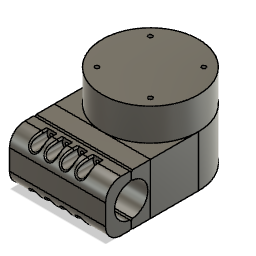
LIDAR Model Stand (Autodesk Fusion 360 design; units mm, degrees)
Autodesk Fusion 360 part; units mm, degrees
box "BoxPrimitive1" add length 75 width 75 height 55 placed x (0, 1, 0) y (-1, 0, 0) z (0, 0, 1) at (70, 0, 0) makes body 1
move_face "OffsetFaces3" offset -15 1 faces at (20, 25, 0) on bodies 1
sketch "Sketch4" plane through (0, 0, 0) normal (1, 0, 0) x (0, 0, -1)
  circle A0 centre (-35, -15) radius 13
  circle A1 centre (-35, -15) radius 20
  line L0 (-55, 0) -> (-55, -15)
  line L1 (-15.0241, -0.1224) -> (-15, -15)
  line L2 (-55, -15) -> (-15, -15)
  line L3 (-15.0241, -0.1224) -> (-55, 0)
  point P0 (-55, 0)
  dimension "d13" = 26
  dimension "d14" = 40
  constraint concentric A0 A1
  constraint vertical L0
  constraint coincident A1 L0.end
  constraint tangent A1 L0
  constraint coincident A1 L1.end
  constraint perpendicular L0 L2
  measures "d13" diameter of A0
  measures "d14" diameter of A1
extrude "Extrude3" add sketch "Sketch4" along normal blind 70 contours A1 L1 L3 | A0 A1 L2 L3 | A1 L0 L3 bodies 1
sketch "Sketch5" plane through (0, -15, 0) normal (0, -1, 0) x (1, 0, 0)
  line L0 (0, 55) -> (0, 48)
  line L1 (0, 48) -> (70, 48)
  line L2 (70, 48) -> (70, 55)
  line L3 (70, 55) -> (0, 55)
  line L4 (0, 51.5) -> (70, 51.5) construction
  circle A0 centre (12, 51.5) radius 1.1
  circle A1 centre (24, 51.5) radius 1.1
  circle A2 centre (36, 51.5) radius 1.1
  circle A3 centre (48, 51.5) radius 1.1
  line L5 (0, 48) -> (60, 48)
  line L6 (60, 48) -> (60, 35)
  line L7 (60, 35) -> (0, 35)
  line L8 (0, 35) -> (0, 48)
  circle A4 centre (12, 18.5) radius 1.1
  circle A5 centre (24, 18.5) radius 1.1
  circle A6 centre (36, 18.5) radius 1.1
  circle A7 centre (48, 18.5) radius 1.1
  dimension "d18" = 12
  dimension "d19" = 12
  dimension "d20" = 12
  dimension "d21" = 12
  dimension "d22" = 2.2
  dimension "d23" = 60
  dimension "d24" = 13
  constraint midpoint L0 L4.start
  constraint midpoint L2 L4.end
  constraint coincident L4 A0.centre
  constraint coincident L4 A1.centre
  constraint coincident L4 A2.centre
  constraint coincident L4 A3.centre
  constraint equal A1 A2
  constraint equal A2 A3
  constraint equal A0 A1
  constraint horizontal L5
  constraint vertical L6
  constraint horizontal L7
  constraint vertical L8
  constraint coincident L0.end L1.start
  constraint symmetric A0 L7 A4
  constraint symmetric A1 L7 A5
  constraint symmetric A2 L7 A6
  constraint symmetric A3 L7 A7
  measures "d18" distance of L4.start A0.centre
  measures "d19" distance of A0.centre A1.centre
  measures "d20" distance of A1.centre A2.centre
  measures "d21" distance of A2.centre A3.centre
  measures "d22" diameter of A0
  measures "d23" distance of L0.end L5.end
  measures "d24" distance of L0.end L7.end
extrude "Extrude4" cut sketch "Sketch5" against normal blind 15 contours A0 | A1 | A2 | A3 | A4 | A5 | A6 | A7 bodies 1
chamfer "Chamfer1" distance 1 angle 45 3 edges at (35, -15, 22) (35, -15, 48) (35, -15, 55) on bodies 1
sketch "Sketch6" plane through (0, 0, 0) normal (-1, 0, 0) x (0, 0, 1)
  line L0 (15.0241, -0.1224) -> (15, -15)
  line L1 (15, -15) -> (21, -15)
  line L2 (21, -15) -> (22.0385, -14.0007)
  arc A0 (47.9615, -14.0007) -> (22.0385, -14.0007) centre (35, -15) ccw
  line L3 (47.9615, -14.0007) -> (49, -15)
  line L4 (49, -15) -> (54, -15)
  circle A1 centre (35, -15) radius 13
  circle A2 centre (35, -15) radius 20
  line L5 (15, -15) -> (55, -15)
  line L6 (55, -15) -> (55, -23)
  line L7 (43, -35) -> (27, -35)
  line L8 (15, -23) -> (15, -15)
  arc A3 (15, -23) -> (27, -35) centre (27, -23) ccw
  arc A4 (43, -35) -> (55, -23) centre (43, -23) ccw
  line L9 (54, -15) -> (55, -14)
  line L10 (55, -14) -> (55, 0)
  line L11 (55, 0) -> (15.0241, -0.1224)
  dimension "d29" = 40
  dimension "d30" = 12
  constraint concentric A0 A1
  constraint coincident A0.start A1
  constraint concentric A1 A2
  constraint horizontal L5
  constraint vertical L6
  constraint horizontal L7
  constraint vertical L8
  constraint coincident L0.end L1.start
  constraint tangent A2 L6
  constraint tangent A2 L7
  constraint tangent L7 A3
  constraint tangent L8 A3
  constraint tangent L6 A4
  constraint tangent L7 A4
  constraint equal A3 A4
  measures "d29" diameter of A2
  measures "d30" radius of A3
extrude "Extrude5" add sketch "Sketch6" against normal blind 70 separate body contours L1 L4 A1 A2 L5 | A2 L7 L8 A3 | A2 L6 L7 A4 makes body 2
chamfer "Chamfer3" distance 1 angle 45 4 edges at (35, -15, 22) (35, -15, 55) (35, -15, 48) (35, -15, 15) on bodies 2
chamfer "Chamfer4" distance 1 angle 45 1 edges at (35, -15, 15) on bodies 1
sketch "Sketch7" plane through (0, -15, 0) normal (0, -1, 0) x (1, 0, 0)
  circle A0 centre (24, 51.5) radius 1.1
  circle A1 centre (36, 51.5) radius 1.1
  circle A2 centre (12, 51.5) radius 1.1
  circle A3 centre (48, 51.5) radius 1.1
  line L0 (70, 54) -> (0, 54)
  line L1 (0, 54) -> (0, 49)
  line L2 (0, 49) -> (70, 49)
  line L3 (70, 49) -> (70, 54)
sketch "Sketch8" plane through (0, -15, 0) normal (0, -1, 0) x (1, 0, 0)
  circle A0 centre (36, 18.5) radius 1.1
  circle A1 centre (24, 18.5) radius 1.1
  circle A2 centre (48, 18.5) radius 1.1
  circle A3 centre (12, 18.5) radius 1.1
  line L0 (0, 16) -> (70, 16)
  line L1 (70, 16) -> (70, 21)
  line L2 (70, 21) -> (0, 21)
  line L3 (0, 21) -> (0, 16)
extrude "Extrude6" cut sketch "Sketch8" sketch "Sketch7" along normal blind 23 contours A0 | A1 | A2 | A3 of sketch 2 contours A0 | A1 | A2 | A3 bodies 2
sketch "Sketch9" plane through (0, -15, 0) normal (0, 1, 0) x (-1, 0, 0)
  circle A0 centre (-24, 51.5) radius 1.1
  circle A1 centre (-36, 51.5) radius 1.1
  circle A2 centre (-12, 51.5) radius 1.1
  circle A3 centre (-48, 51.5) radius 1.1
  line L0 (-70, 49) -> (0, 49)
  line L1 (0, 49) -> (0, 54)
  line L2 (0, 54) -> (-70, 54)
  line L3 (-70, 54) -> (-70, 49)
  circle A4 centre (-12, 51.5) radius 3.75
  circle A5 centre (-24, 51.5) radius 3.75
  circle A6 centre (-36, 51.5) radius 3.75
  circle A7 centre (-48, 51.5) radius 3.75
  circle A8 centre (-12, 18.5) radius 3.75
  circle A9 centre (-24, 18.5) radius 3.75
  circle A10 centre (-36, 18.5) radius 3.75
  circle A11 centre (-48, 18.5) radius 3.75
  dimension "d37" = 7.5
  dimension "d40" = -36
  dimension "d41" = -33
  constraint concentric A2 A4
  measures "d37" diameter of A4
extrude "Extrude7" cut sketch "Sketch9" against normal blind 36 from surface at -4 contours L0 L2 A7 | L0 A7 | L2 A7 | L0 L2 A6 | L0 A6 | L2 A6 | L0 L2 A5 | L0 A5 | L2 A5 | L0 L2 A4 | L0 A4 | L2 A4 | A8 | A9 | A10 | A11 bodies 2
fillet "Fillet1" radius 1 24 edges at (46.6537, -21, 15) (48, -34.0199, 22.25) (49.3463, -21, 15) (34.6537, -21, 15) (36, -34.0199, 22.25) (37.3463, -21, 15) (22.6537, -21, 15) (24, -34.0199, 22.25) (25.3463, -21, 15) (10.6537, -21, 15) (12, -34.0199, 22.25) (13.3463, -21, 15) (49.3463, -21, 55) (48, -34.0199, 47.75) (46.6537, -21, 55) (37.3463, -21, 55) (36, -34.0199, 47.75) (34.6537, -21, 55) (25.3463, -21, 55) (24, -34.0199, 47.75) (22.6537, -21, 55) (13.3463, -21, 55) (12, -34.0199, 47.75) (10.6537, -21, 55) on bodies 2
move_face "OffsetFaces1" offset -0.4 8 faces at (13.0945, -17.6667, 18.6095) (24.8768, -16.3333, 19.1642) (35.034, -16.3333, 19.0261) (48.5018, -16.3333, 19.4789) (49.0986, -17.6667, 51.4452) (37.0986, -17.6667, 51.4452) (25.0986, -17.6667, 51.4452) (13.0986, -17.6667, 51.4452) on bodies 2
move_face "OffsetFaces4" offset 5 1 faces at (0, -8.0766, 52.3644) on bodies 1
move_face "OffsetFaces5" offset 5 1 faces at (0, -32.6667, 35) on bodies 2
move_body "Move1" bodies 2 1 to x (1, 0, 0) y (0, 0, -1) z (0, 1, 0) at (0, -70.5, 32.5)
sketch "Sketch18" plane through (0, -15.5, 0) normal (0, 1, 0) x (-1, 0, 0)
  line L0 (-70, -42.5) -> (5, -42.5)
  line L1 (5, -42.5) -> (5, 32.5)
  line L2 (5, 32.5) -> (-70, 32.5)
  line L3 (-70, 32.5) -> (-70, -42.5)
  line L4 (5, -42.5) -> (-70, 32.5) construction
  line L5 (5, 32.5) -> (-70, -42.5) construction
  circle A0 centre (-32.5, -5) radius 37.5
  dimension "d75" = 75
  constraint coincident L0.end L1.start
  constraint coincident L2.end L3.start
  constraint coincident L1.end L2.start
  constraint coincident L0.start L3.end
  constraint midpoint L4 A0.centre
  measures "d75" diameter of A0
extrude "Extrude17" add sketch "Sketch18" along normal blind 25 separate body contours A0 makes body 3
extrude "Extrude16" cut sketch "Sketch18" against normal blind 40 contours L0 L1 A0 bodies 1
extrude "Extrude15" cut sketch "Sketch18" against normal blind 40 contours L0 L3 A0 bodies 1
sketch "Sketch19" plane through (0, -55.5, 0) normal (0, -1, 0) x (1, 0, 0)
  arc A0 (-5, -5) -> (70, -5) centre (32.5, -5) ccw
  line L0 (70, -5) -> (70, 32.5)
  line L1 (70, 32.5) -> (-5, 32.5)
  line L2 (-5, 32.5) -> (-5, -5)
  circle A1 centre (32.5, -5) radius 32.5
  dimension "d82" = 65
  constraint concentric A0 A1
  measures "d82" diameter of A1
extrude "Extrude18" cut sketch "Sketch19" against normal up to surface (62 mm away) contours A1 bodies 1 3
sketch "Sketch20" plane through (0, 6.5, 0) normal (0, -1, 0) x (1, 0, 0)
  circle A0 centre (32.5, -5) radius 32.5
  line L0 (32.5, -5) -> (32.5, 15.86) construction
  line L1 (32.5, 15.86) -> (53.36, 15.86) construction
  circle A1 centre (53.36, 15.86) radius 1.6
  line L2 (32.5, -5) -> (50, -5) construction
  circle A2 centre (53.36, -25.86) radius 1.6
  circle A3 centre (11.64, 15.86) radius 1.6
  circle A4 centre (11.64, -25.86) radius 1.6
  dimension "d88" = 20.86
  dimension "d89" = 20.86
  dimension "d90" = 3.2
  constraint coincident A0.centre L0.start
  constraint vertical L0
  constraint horizontal L1
  constraint coincident L1.end A1.centre
  constraint perpendicular L0 L2
  constraint symmetric A1 L2 A2
  constraint symmetric L0 A1 A3
  constraint symmetric L2 A3 A4
  measures "d88" distance of A0.centre L0.end
  measures "d89" distance of L0.end L1.end
  measures "d90" diameter of A1
extrude "Extrude19" cut sketch "Sketch20" against normal blind 3 contours A1 | A2 | A3 | A4 bodies 3
fillet "Fillet4" radius 1.5 1 edges at (2.1994, -55.5, 6.7525) on bodies 1
